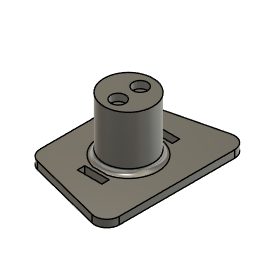
Magnetic Lock v7 (Autodesk Fusion 360 design; units mm, degrees)
Autodesk Fusion 360 part; units mm, degrees
sketch "Sketch1" plane through (0, 0, 0) normal (0, 1, 0) x (1, 0, 0)
  line L0 (46.0121, 0.2) -> (46.0121, -59.8)
  line L1 (6.0121, -29.5532) -> (6.0121, -9.5532)
  line L2 (6.0121, -29.5532) -> (6.0121, -49.5532)
  line L3 (6.0121, -9.5532) -> (46.0121, 0.2)
  line L4 (6.0121, -49.5532) -> (46.0121, -59.8)
  line L5 (31.0121, -13.6532) -> (21.0121, -13.6532)
  line L6 (21.0121, -13.6532) -> (21.0121, -16.6532)
  line L7 (21.0121, -16.6532) -> (31.0121, -16.6532)
  line L8 (31.0121, -16.6532) -> (31.0121, -13.6532)
  line L9 (31.0121, -42.4532) -> (21.0121, -42.4532)
  line L10 (21.0121, -42.4532) -> (21.0121, -45.4532)
  line L11 (21.0121, -45.4532) -> (31.0121, -45.4532)
  line L12 (31.0121, -45.4532) -> (31.0121, -42.4532)
  point P0 (26.0121, -15.0532)
  point P1 (25.8317, -44.4989)
  dimension "d1" = 60
  dimension "d6" = 20
  dimension "d7" = 20
  dimension "d9" = 40
  dimension "d10" = 40
  dimension "d11" = 20
  dimension "d12" = 14.5
  dimension "d13" = 10
  dimension "d14" = 3
  dimension "d15" = 10
  dimension "d16" = 3
  dimension "d19" = 12.9
  dimension "d20" = 12.9
  dimension "d21" = 25.8
  dimension "d22" = 15
  dimension "d23" = 15
  constraint parallel L0 L1
  constraint parallel L1 L2
  constraint horizontal L5
  constraint perpendicular L5 L6
  constraint parallel L5 L7
  constraint parallel L6 L8
  constraint horizontal L9
  constraint perpendicular L9 L10
  constraint parallel L9 L11
  constraint parallel L10 L12
  measures "d1" distance of L0.start L0.end
  measures "d6" distance of L1.start L1.end
  measures "d7" distance of L1.start L2.end
  measures "d9" distance of L0 L2
  measures "d10" distance of L1.end L2.end
  measures "d11" distance of L0 P0
  measures "d12" vertical distance of L1.start P0
  measures "d13" distance of L6.end L7.end
  measures "d14" distance of L5.end L6.end
  measures "d15" distance of L10.end L11.end
  measures "d16" distance of L9.end L10.end
  measures "d19" distance of L1.start L9
  measures "d20" vertical distance of L1.start L6.end
  measures "d21" distance of L7 L9
  measures "d22" distance of L2 L10
  measures "d23" distance of L1 L6
extrude "Extrude1" add sketch "Sketch1" along normal blind 3
sketch "Sketch2" plane through (0, 3, 0) normal (0, 1, 0) x (-1, 0, 0)
  line L0 (-31.0121, 42.4532) -> (-31.0121, 45.4532)
  line L1 (-31.0121, 45.4532) -> (-21.0121, 45.4532)
  line L2 (-21.0121, 45.4532) -> (-21.0121, 42.4532)
  line L3 (-21.0121, 42.4532) -> (-31.0121, 42.4532)
  line L4 (-31.0121, 13.6532) -> (-31.0121, 16.6532)
  line L5 (-31.0121, 16.6532) -> (-21.0121, 16.6532)
  line L6 (-21.0121, 16.6532) -> (-21.0121, 13.6532)
  line L7 (-21.0121, 13.6532) -> (-31.0121, 13.6532)
  line L8 (-6.0121, 9.5532) -> (-6.0121, 49.5532)
  line L9 (-6.0121, 49.5532) -> (-46.0121, 59.8)
  line L10 (-46.0121, 59.8) -> (-46.0121, -0.2)
  line L11 (-46.0121, -0.2) -> (-6.0121, 9.5532)
  circle A0 centre (-26.0121, 29.5532) radius 10
  point P0 (-26.0121, 29.5532)
  dimension "d38" = 12.9
  dimension "d39" = 12.9
  dimension "d42" = 20
  constraint coincident P0 A0.centre
  measures "d38" distance of L3 P0
  measures "d39" distance of L5 P0
  measures "d42" diameter of A0
extrude "Extrude2" add sketch "Sketch2" along normal blind 22 contours A0
sketch "Sketch3" plane through (0, 25, 0) normal (0, 1, 0) x (-1, 0, 0)
  line L0 (-28.0121, 38.7532) -> (-24.0121, 38.7532)
  line L1 (-24.0121, 38.7532) -> (-24.0121, 20.7532)
  line L2 (-24.0121, 20.7532) -> (-28.0121, 20.7532)
  line L3 (-28.0121, 20.7532) -> (-28.0121, 38.7532)
  line L4 (-28.0121, 38.7532) -> (-24.0121, 20.7532) construction
  line L5 (-24.0121, 38.7532) -> (-28.0121, 20.7532) construction
  circle A0 centre (-26.0121, 29.5532) radius 10
  point P0 (-26.0121, 29.7532)
  dimension "d28" = 18
  constraint horizontal L0
  constraint perpendicular L0 L1
  constraint parallel L0 L2
  constraint parallel L1 L3
  constraint coincident L4 P0
  constraint coincident L5 P0
  measures "d28" distance of L0.end L1.end
fillet "Fillet4" radius 2 1 edges at (35.3354, 3, 33.1694)
fillet "Fillet3" radius 5 4 edges at (6.0121, 1.5, 9.5532) (6.0121, 1.5, 49.5532) (46.0121, 1.5, 59.8) (46.0121, 1.5, -0.2)
sketch "Sketch5" plane through (0, 25, 0) normal (0, 1, 0) x (-1, 0, 0)
  circle A0 centre (-26.0121, 29.5532) radius 10
  circle A1 centre (-26.282, 34.0532) radius 2.975
  circle A2 centre (-26.282, 25.0532) radius 2.975
  dimension "d48" = 5.95
  dimension "d49" = 5.95
  dimension "d50" = 4.5
  dimension "d51" = 4.5
  measures "d48" diameter of A1
  measures "d49" diameter of A2
  measures "d50" vertical distance of A0.centre A1.centre
  measures "d51" vertical distance of A0.centre A2.centre
extrude "Extrude5" cut sketch "Sketch5" against normal blind 2.93 contours A1 | A2
sketch "Sketch6" plane through (0, 3, 0) normal (0, 1, 0) x (-1, 0, 0)
  arc A0 (-46.0121, 6.1656) -> (-39.8276, 1.308) centre (-41.0121, 6.1656) ccw
  line L0 (-39.8276, 1.308) -> (-9.8276, 8.6229)
  arc A1 (-9.8276, 8.6229) -> (-6.0121, 13.4806) centre (-11.0121, 13.4806) ccw
  line L1 (-6.0121, 13.4806) -> (-6.0121, 45.6726)
  arc A2 (-6.0121, 45.6726) -> (-9.7713, 50.5162) centre (-11.0121, 45.6726) ccw
  line L2 (-9.7713, 50.5162) -> (-39.7713, 58.2013)
  arc A3 (-39.7713, 58.2013) -> (-46.0121, 53.3577) centre (-41.0121, 53.3577) ccw
  line L3 (-46.0121, 53.3577) -> (-46.0121, 6.1656)
  line L4 (-31.0121, 42.4532) -> (-31.0121, 45.4532)
  line L5 (-31.0121, 45.4532) -> (-21.0121, 45.4532)
  line L6 (-21.0121, 45.4532) -> (-21.0121, 42.4532)
  line L7 (-21.0121, 42.4532) -> (-31.0121, 42.4532)
  line L8 (-31.0121, 13.6532) -> (-31.0121, 16.6532)
  line L9 (-31.0121, 16.6532) -> (-21.0121, 16.6532)
  line L10 (-21.0121, 16.6532) -> (-21.0121, 13.6532)
  line L11 (-21.0121, 13.6532) -> (-31.0121, 13.6532)
  circle A4 centre (-26.0121, 29.5532) radius 12
  line L12 (-21.0121, 17.9232) -> (-31.0121, 17.9232)
  line L13 (-31.0121, 17.9232) -> (-31.0121, 12.3832)
  line L14 (-31.0121, 12.3832) -> (-21.0121, 12.3832)
  line L15 (-21.0121, 12.3832) -> (-21.0121, 17.9232)
  line L16 (-21.0121, 17.9232) -> (-31.0121, 12.3832) construction
  line L17 (-31.0121, 17.9232) -> (-21.0121, 12.3832) construction
  line L18 (-31.0121, 41.1832) -> (-21.0121, 41.1832)
  line L19 (-21.0121, 41.1832) -> (-21.0121, 46.7232)
  line L20 (-21.0121, 46.7232) -> (-31.0121, 46.7232)
  line L21 (-31.0121, 46.7232) -> (-31.0121, 41.1832)
  line L22 (-31.0121, 41.1832) -> (-21.0121, 46.7232) construction
  line L23 (-21.0121, 41.1832) -> (-31.0121, 46.7232) construction
  point P0 (-26.0121, 15.1532)
  point P1 (-26.0121, 43.9532)
  dimension "d52" = 10
  dimension "d53" = 5.54
  dimension "d54" = 5.54
  constraint horizontal L12
  constraint perpendicular L12 L13
  constraint parallel L12 L14
  constraint parallel L13 L15
  constraint coincident L16 P0
  constraint coincident L17 P0
  constraint horizontal L18
  constraint perpendicular L18 L19
  constraint parallel L18 L20
  constraint parallel L19 L21
  constraint coincident L22 P1
  constraint coincident L23 P1
  measures "d52" distance of L13.end L14.end
  measures "d53" distance of L12.end L13.end
  measures "d54" distance of L18.end L19.end
extrude "Extrude6" cut sketch "Sketch6" along normal blind 11 contours L7 A4 L18 L19 L21 | A4 L18 | A4 L12 | L9 A4 L12 L13 L15
equation "d12 = ( 29 / 2 ) * 1 mm"
equation "d26 = 37 mm - 10 mm - 5 mm"
